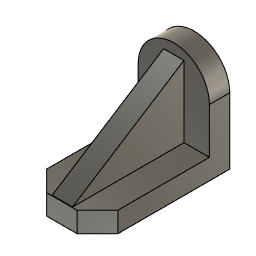
A1 (Autodesk Fusion 360 design; units mm, degrees)
Autodesk Fusion 360 part; units mm, degrees
sketch "Sketch1" plane through (0, 0, 0) normal (0, 0, 1) x (1, 0, 0)
  line L0 (-30, 50) -> (12, 50)
  line L1 (12, 50) -> (12, -16)
  line L2 (12, -16) -> (-30, -16)
  line L3 (-30, -16) -> (-30, 50)
  dimension "d1" = 42
  dimension "d2" = 66
  constraint horizontal L0
  constraint vertical L1
  constraint horizontal L2
  constraint vertical L3
  measures "d1" distance of L0.start L0.end
  measures "d2" distance of L0.start L2.end
extrude "Extrude1" add sketch "Sketch1" along normal blind 12
sketch "Sketch2" plane through (0, 0, 0) normal (0, 0, 1) x (1, 0, 0)
  line L0 (-30, 50) -> (12, 50)
  line L1 (12, 50) -> (12, 62)
  line L2 (12, 62) -> (-30, 62)
  line L3 (-30, 62) -> (-30, 50)
  dimension "d5" = 42
  dimension "d6" = 12
  constraint horizontal L0
  constraint vertical L1
  constraint horizontal L2
  constraint vertical L3
  measures "d5" distance of L0.start L0.end
  measures "d6" distance of L0.start L2.end
extrude "Extrude2" add sketch "Sketch2" along normal blind 39
sketch "Sketch3" plane through (0, 0, 0) normal (0, 0, 1) x (1, 0, 0)
sketch "Sketch4" plane through (0, 0, 0) normal (0, 0, 1) x (1, 0, 0)
sketch "Sketch5" plane through (0, 0, 0) normal (0, 1, 0) x (1, 0, 0)
sketch "Sketch6" plane through (0, 50, 0) normal (0, -1, 0) x (1, 0, 0)
  line L0 (-30, 12) -> (12, 12)
  line L1 (12, 12) -> (12, 39)
  line L2 (12, 39) -> (-30, 39)
  line L3 (-30, 39) -> (-30, 12)
  arc A0 (12, 39) -> (-30, 39) centre (-9, 39) ccw
  constraint coincident L1.end L2.start
  constraint coincident L2.end L3.start
  constraint tangent L3 A0
extrude "Extrude3" add sketch "Sketch6" against normal blind 12 contours L2 A0
sketch "Sketch7" plane through (0, 0, 12) normal (0, 0, 1) x (-1, 0, 0)
  line L0 (30, 16) -> (-12, 16)
  line L1 (-12, 16) -> (-12, -50)
  line L2 (-12, -50) -> (30, -50)
  line L3 (30, -50) -> (30, 16)
form "Form1" [no effect]
sketch "Sketch13" plane through (0, 0, 12.0166) normal (0, 0, 1) x (1, 0, 0)
sketch "Sketch14" plane through (0, 0, 12) normal (0, 0, 1) x (1, 0, 0)
sketch "Sketch15" plane through (0, 0, 0) normal (1, 0, 0) x (0, 1, 0)
form "Form2" [no effect]
sketch "Sketch16" plane through (0, 0, 0) normal (1, 0, 0) x (0, 1, 0)
  line L0 (-15.7632, 12.0147) -> (50, 12.0147)
  line L1 (50, 12.0147) -> (-16, 12.0147)
  line L2 (50, 12.0147) -> (50, 54.0147)
  line L3 (50, 54.0147) -> (-15.7632, 12.0147)
  dimension "d17" = 66
  dimension "d18" = 42
  constraint horizontal L0
  constraint parallel L0 L1
  constraint perpendicular L0 L2
  measures "d17" distance of L0.end L1.end
  measures "d18" distance of L0.end L2.end
extrude "Extrude6" add sketch "Sketch16" along normal blind -3 and the other way blind 15
sketch "Sketch17" plane through (0, 0, 0) normal (0, 0, 1) x (1, 0, 0)
sketch "Sketch18" plane through (0, 0, 12) normal (0, 0, 1) x (1, 0, 0)
  line L0 (12, -16) -> (0, -16)
  line L1 (0, -16) -> (12, -4)
  line L2 (12, -4) -> (12, -16)
  line L3 (-30, -16) -> (-18, -16)
  line L4 (-18, -16) -> (-30, -4)
  line L5 (-30, -4) -> (-30, -16)
  constraint horizontal L0
  constraint perpendicular L0 L2
  constraint perpendicular L2 L3
  constraint perpendicular L1 L4
  constraint perpendicular L0 L5
extrude "Extrude7" cut sketch "Sketch18" against normal blind 12 contours L0 L1 L2
extrude "Extrude8" cut sketch "Sketch18" against normal blind 12 contours L3 L4 L5
named bodies: "A1"
